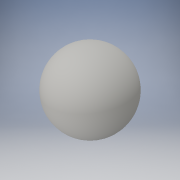
# Autodesk Inventor part: BOULDER
Saved by Autodesk Inventor 2016 (Build 200138000, 138)
## iProperties
Created: 2016-01-10
Part Number: BOULDER
Material: Generic
Document SubType Name: Modeling
Designer: hartc3
Density: 1 g/cm^3
Appearance: Default
Author: hartc3
Autodesk Inventor part; units mm, degrees
ref_plane "YZ Plane" through (0, 0, 0) normal (1, 0, 0) x (0, 1, 0)
ref_plane "XZ Plane" through (0, 0, 0) normal (0, 1, 0) x (-1, 0, 0)
ref_plane "XY Plane" through (0, 0, 0) normal (0, 0, 1) x (1, 0, 0)
sketch "Sketch1" plane through (0, 0, 0) normal (1, 0, 0) x (0, 1, 0)
  arc A0 (-127, 0) -> (127, 0) centre (0, 0) ccw
  line L0 (127, 0) -> (-127, 0)
  dimension "d1" = 254
  constraints: 2 end point, 2 point on circle, 1 centre point, 1 coincident, 1 horizontal
  measures "d1" diameter of A0
revolve "Revolution1" add sketch "Sketch1" angle 360 about axis through (0, 127, 0) along (0, -1, 0)
body "Solid1"
